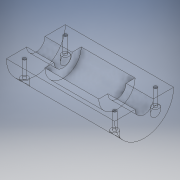
# Autodesk Inventor part: Slider Mount_D2
Saved by Autodesk Inventor 2018 (Build 220112000, 112)
## iProperties
Created: 2018-01-08
Part Number: Slider Mount_D2
Material: Generic
Document SubType Name: Modeling
Designer: njcfu
Density: 1 g/cm^3
Appearance: Default
Author: njcfu
Autodesk Inventor part; units mm, degrees
ref_plane "YZ Plane" through (0, 0, 0) normal (1, 0, 0) x (0, 1, 0)
ref_plane "XZ Plane" through (0, 0, 0) normal (0, 1, 0) x (-1, 0, 0)
ref_plane "XY Plane" through (0, 0, 0) normal (0, 0, 1) x (1, 0, 0)
sketch "Sketch2" plane through (0, 0, 0) normal (1, 0, 0) x (0, 1, 0)
  arc A0 (0, 25.4) -> (0, -25.4) centre (0, 0) ccw
  arc A1 (0, 41.275) -> (0, -41.275) centre (0, 0) ccw
  line L0 (0, 41.275) -> (0, 25.4)
  line L1 (0, -25.4) -> (0, -41.275)
  dimension "d0" = 25.4
  dimension "d2" = 15.875
  dimension "d68" = 41.275
  constraints: 4 end point, 4 point on circle, 2 centre point, 2 coincident, 2 point on line, 1 vertical
  measures "d0" radius of A0
  measures "d2" distance of L0.start L0.end
  measures "d68" radius of A1
extrude "Extrusion1" add sketch "Sketch2" along normal mid plane 75.3999
sketch "Sketch3" plane through (37.7, 0, 0) normal (1, 0, 0) x (0, 0, -1)
  arc A0 (-12.7, 0) -> (12.7, 0) centre (0, 0) ccw
  arc A1 (-41.275, 0) -> (41.275, 0) centre (0, 0) ccw
  line L0 (-12.7, 0) -> (-41.275, 0)
  line L1 (12.7, 0) -> (41.275, 0)
  dimension "d5" = 12.7
  dimension "d7" = 28.575
  dimension "d8" = 28.575
  dimension "d70" = 41.275
  constraints: 4 end point, 4 point on circle, 2 centre point, 2 coincident, 1 horizontal, 1 point on line
  measures "d5" radius of A0
  measures "d7" distance of L0.start L0.end
  measures "d8" distance of L1.start L1.end
  measures "d70" radius of A1
extrude "Extrusion2" add sketch "Sketch3" along normal blind 38.1
sketch "Sketch4" plane through (-37.7, 0, 0) normal (-1, 0, 0) x (0, 0, 1)
  arc A0 (-12.7, 0) -> (12.7, 0) centre (0, 0) ccw
  arc A1 (-41.275, 0) -> (41.275, 0) centre (0, 0) ccw
  line L0 (-12.7, 0) -> (-41.275, 0)
  line L1 (12.7, 0) -> (41.275, 0)
  point P0 (0, 0)
  dimension "d11" = 12.7
  dimension "d13" = 28.575
  dimension "d14" = 28.575
  dimension "d15" = 12.7
  dimension "d16" = 12.7
  dimension "d69" = 41.275
  constraints: 4 end point, 4 point on circle, 2 centre point, 2 coincident, 1 horizontal, 1 point on line
  measures "d11" radius of A0
  measures "d13" distance of L0.start L0.end
  measures "d14" distance of L1.start L1.end
  measures "d15" distance of point (0, 0) L0.start
  measures "d16" distance of L1.start point (0, 0)
  measures "d69" radius of A1
extrude "Extrusion3" add sketch "Sketch4" along normal blind 38.1
sketch "Sketch6" plane through (37.7, 0, -12.7) normal (0, 1, 0) x (1, 0, 0)
  circle A0 centre (-100.7999, 15.875) radius 2.413
  circle A1 centre (25.4, 15.875) radius 2.413
  circle A2 centre (25.4, -41.275) radius 2.413
  circle A3 centre (-100.7999, -41.275) radius 2.413
  line L0 (-113.4999, 28.575) -> (38.1, 28.575) projected
  line L1 (-113.4999, 0) -> (-113.4999, 28.575) projected
  line L2 (38.1, 28.575) -> (38.1, 0) projected
  line L3 (38.1, -25.4) -> (38.1, -53.975) projected
  line L4 (38.1, -53.975) -> (-113.4999, -53.975) projected
  line L5 (-113.4999, -53.975) -> (-113.4999, -25.4) projected
  point P0 (-37.7, -12.7)
  dimension "d45" = 12.7
  dimension "d46" = 12.7
  dimension "d47" = 12.7
  dimension "d48" = 12.7
  dimension "d49" = 12.7
  dimension "d50" = 12.7
  dimension "d51" = 12.7
  dimension "d52" = 12.7
  dimension "d53" = 4.826
  dimension "d54" = 4.826
  dimension "d55" = 4.826
  dimension "d56" = 4.826
  constraints: 4 centre point
  measures "d45" distance from line of L0 A0.centre
  measures "d46" distance from line of L1 A0.centre
  measures "d47" distance from line of L2 A1.centre
  measures "d48" distance from line of L0 A1.centre
  measures "d49" distance from line of L3 A2.centre
  measures "d50" distance from line of A2.centre L4
  measures "d51" distance from line of L4 A3.centre
  measures "d52" distance from line of L5 A3.centre
  measures "d53" diameter of A0
  measures "d54" diameter of A1
  measures "d55" diameter of A2
  measures "d56" diameter of A3
extrude "Extrusion4" cut sketch "Sketch6" against normal blind 38.1
ref_plane "Work Plane1" through (37.7, -28.4375, -12.7) normal (0, 1, 0) x (1, 0, 0)
sketch "Sketch7" plane through (37.7, -28.4375, -12.7) normal (0, 1, 0) x (1, 0, 0)
  circle A0 centre (25.4, 15.875) radius 5.08
  circle A1 centre (25.4, -41.275) radius 5.08
  circle A2 centre (-100.7999, -41.275) radius 5.08
  circle A3 centre (-100.7999, 15.875) radius 5.08
  circle A4 centre (25.4, -41.275) radius 2.413 projected
  circle A5 centre (25.4, 15.875) radius 2.413 projected
  circle A6 centre (-100.7999, 15.875) radius 2.413 projected
  circle A7 centre (-100.7999, -41.275) radius 2.413 projected
  point P0 (-37.7, -12.7)
  dimension "d60" = 10.16
  dimension "d61" = 10.16
  dimension "d62" = 10.16
  dimension "d63" = 10.16
  constraints: 4 centre point, 4 concentric
  measures "d60" diameter of A0
  measures "d61" diameter of A1
  measures "d62" diameter of A3
  measures "d63" diameter of A2
extrude "Extrusion5" cut sketch "Sketch7" along normal blind 5.08 and the other way blind 12.7
body "Solid1"
